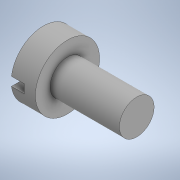
# Autodesk Inventor part: M2x4
Saved by Autodesk Inventor 2021 (Build 250183000, 183)
## iProperties
Created: 2024-03-24
Part Number: M2x4
Material: Generic
Document SubType Name: Modeling
Designer: Lukas
Density: 1 g/cm^3
Appearance: Default
Author: Lukas
Autodesk Inventor part; units mm, degrees
ref_plane "YZ Plane" through (0, 0, 0) normal (1, 0, 0) x (0, 1, 0)
ref_plane "XZ Plane" through (0, 0, 0) normal (0, 1, 0) x (-1, 0, 0)
ref_plane "XY Plane" through (0, 0, 0) normal (0, 0, 1) x (1, 0, 0)
sketch "Sketch1" plane through (0, 0, 0) normal (0, 0, 1) x (1, 0, 0)
  line L0 (0, 0) -> (-2.7, 0)
  line L1 (-2.7, 0) -> (-2.7, 1.85)
  line L2 (-2.7, 1.85) -> (-1.3, 1.85)
  line L3 (-1.3, 1.85) -> (-1.3, 1)
  line L4 (-1.3, 1) -> (2.7, 1)
  line L5 (2.7, 1) -> (2.7, 0)
  line L6 (2.7, 0) -> (0, 0)
  dimension "d0" = 1
  dimension "d1" = 4
  dimension "d2" = 1.4
  dimension "d3" = 1.85
  constraints: 14 end point, 6 perpendicular, 1 collinear, 1 horizontal, 1 point on line
  measures "d0" distance of L4.end L5.end
  measures "d1" distance of L3.end L4.end
  measures "d2" distance of L1.end L2.end
  measures "d3" distance of L0.end L1.end
revolve "Revolution1" add sketch "Sketch1" angle 360 about axis through (2.7, 0, 0) along (-1, 0, 0)
sketch "Sketch2" plane through (-2.7, 0, 0) normal (-1, 0, 0) x (0, 0, 1)
  line L0 (-2, 0.25) -> (2, 0.25)
  line L1 (2, 0.25) -> (2, -0.25)
  line L2 (2, -0.25) -> (-2, -0.25)
  line L3 (-2, -0.25) -> (-2, 0.25)
  point P0 (0, 0)
  point P1 (-2, 0)
  point P2 (0, 0.25)
  dimension "d5" = 0.5
  dimension "d6" = 4
  constraints: 8 end point, 2 midpoint, 2 parallel, 1 horizontal, 1 horizontal alignment, 1 perpendicular, 1 vertical alignment
  measures "d5" distance of L2.end L0.start
  measures "d6" distance of L0.start L0.end
extrude "Extrusion1" cut sketch "Sketch2" against normal blind 0.75
body "Solid1"
